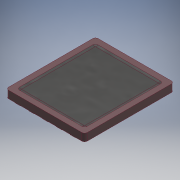
# Autodesk Inventor part: Semiconductor_RadiationDiode
Saved by Autodesk Inventor 2017 (Build 210142000, 142)
## iProperties
Created: 2018-01-16
Part Number: Semiconductor_RadiationDiode
Material: ABS Plastic
Document SubType Name: Modeling
Designer: Bradley
Mass: 0.33228 g
Surface Area: 5.66161 cm^2
Volume: 0.313472 cm^3
Density: 1.06 g/cm^3
Appearance: Smooth - Dark Maroon
Stock Number: X100-7 SMD
Author: Bradley
Autodesk Inventor part; units mm, degrees
ref_plane "YZ Plane" through (0, 0, 0) normal (1, 0, 0) x (0, 1, 0)
ref_plane "XZ Plane" through (0, 0, 0) normal (0, 1, 0) x (-1, 0, 0)
ref_plane "XY Plane" through (0, 0, 0) normal (0, 0, 1) x (1, 0, 0)
sketch "Sketch1" plane through (0, 0, 0) normal (0, 0, 1) x (1, 0, 0)
  line L0 (-7.25, -8.25) -> (7.25, -8.25)
  line L1 (7.25, -8.25) -> (7.25, 8.25)
  line L2 (7.25, 8.25) -> (-7.25, 8.25)
  line L3 (-7.25, 8.25) -> (-7.25, -8.25)
  line L4 (-7.25, -8.25) -> (7.25, 8.25) construction
  line L5 (7.25, -8.25) -> (-7.25, 8.25) construction
  point P0 (0, 0)
  dimension "d0" = 14.5
  dimension "d1" = 16.5
  constraints: 12 end point, 2 midpoint, 2 parallel, 1 horizontal, 1 perpendicular
  measures "d0" distance of L2.end L1.end
  measures "d1" distance of L1.end L0.end
extrude "Extrusion1" add sketch "Sketch1" along normal mid plane 1.38
fillet "Fillet1" radius 0.5 4 edges at (-7.25, 8.25, 0) (7.25, 8.25, 0) (7.25, -8.25, 0) (-7.25, -8.25, 0)
sketch "Sketch2" plane through (0, 0, 0.69) normal (0, 0, 1) x (1, 0, 0)
  arc A0 (-7.25, -7.75) -> (-6.75, -8.25) centre (-6.75, -7.75) ccw projected
  line L0 (-6.75, -8.25) -> (6.75, -8.25) projected
  arc A1 (6.75, -8.25) -> (7.25, -7.75) centre (6.75, -7.75) ccw projected
  line L1 (7.25, -7.75) -> (7.25, 7.75) projected
  arc A2 (7.25, 7.75) -> (6.75, 8.25) centre (6.75, 7.75) ccw projected
  line L2 (6.75, 8.25) -> (-6.75, 8.25) projected
  arc A3 (-6.75, 8.25) -> (-7.25, 7.75) centre (-6.75, 7.75) ccw projected
  line L3 (-7.25, 7.75) -> (-7.25, -7.75) projected
  line L4 (5.75, -7.25) -> (-5.75, -7.25)
  line L5 (-6.25, -6.75) -> (-6.25, 6.75)
  line L6 (-5.75, 7.25) -> (5.75, 7.25)
  line L7 (6.25, 6.75) -> (6.25, -6.75)
  line L8 (6.25, -7.25) -> (-6.25, 7.25) construction
  line L9 (-6.25, -7.25) -> (6.25, 7.25) construction
  arc A4 (-5.75, 7.25) -> (-6.25, 6.75) centre (-5.75, 6.75) ccw
  arc A5 (6.25, 6.75) -> (5.75, 7.25) centre (5.75, 6.75) ccw
  arc A6 (5.75, -7.25) -> (6.25, -6.75) centre (5.75, -6.75) ccw
  arc A7 (-6.25, -6.75) -> (-5.75, -7.25) centre (-5.75, -6.75) ccw
  point P0 (0, 0)
  dimension "d5" = 1
  dimension "d6" = 1
  dimension "d7" = 0.5
  constraints: 12 end point, 8 point on circle, 8 point on line, 8 tangent, 4 centre point, 3 equal radius, 2 midpoint, 2 parallel, 1 horizontal, 1 perpendicular
  measures "d5" distance between parallel lines of L6 L2
  measures "d6" distance between parallel lines of L3 L5
  measures "d7" radius of A4
extrude "Extrusion2" cut sketch "Sketch2" against normal blind 0.1 contours L4 A7 L5 A4 L6 A5 L7 A6
fillet "Fillet2" radius 1 8 edges at (-6.25, 0, 0.59) (-6.1036, 7.1036, 0.59) (0, 7.25, 0.59) (6.1036, 7.1036, 0.59) (6.25, 0, 0.59) (6.1036, -7.1036, 0.59) (0, -7.25, 0.59) (-6.1036, -7.1036, 0.59)
sketch "Sketch3" plane through (0, 0, -0.69) normal (0, 0, -1) x (-1, 0, 0)
  arc A0 (6.75, -8.25) -> (7.25, -7.75) centre (6.75, -7.75) ccw projected
  line L0 (7.25, -7.75) -> (7.25, 7.75) projected
  arc A1 (7.25, 7.75) -> (6.75, 8.25) centre (6.75, 7.75) ccw projected
  line L1 (6.75, 8.25) -> (-6.75, 8.25) projected
  arc A2 (-6.75, 8.25) -> (-7.25, 7.75) centre (-6.75, 7.75) ccw projected
  line L2 (-7.25, 7.75) -> (-7.25, -7.75) projected
  arc A3 (-7.25, -7.75) -> (-6.75, -8.25) centre (-6.75, -7.75) ccw projected
  line L3 (-6.75, -8.25) -> (6.75, -8.25) projected
  line L4 (-5.58, 8.25) -> (-4.58, 8.25)
  line L5 (-4.58, 8.25) -> (-4.58, 6.45)
  line L6 (-4.58, 6.45) -> (-5.58, 6.45)
  line L7 (-5.58, 6.45) -> (-5.58, 8.25)
  line L8 (-3.04, 8.25) -> (-2.04, 8.25)
  line L9 (-2.04, 8.25) -> (-2.04, 6.45)
  line L10 (-2.04, 6.45) -> (-3.04, 6.45)
  line L11 (-3.04, 6.45) -> (-3.04, 8.25)
  line L12 (-0.5, 8.25) -> (0.5, 8.25)
  line L13 (0.5, 8.25) -> (0.5, 6.45)
  line L14 (0.5, 6.45) -> (-0.5, 6.45)
  line L15 (-0.5, 6.45) -> (-0.5, 8.25)
  line L16 (2.04, 8.25) -> (3.04, 8.25)
  line L17 (3.04, 8.25) -> (3.04, 6.45)
  line L18 (3.04, 6.45) -> (2.04, 6.45)
  line L19 (2.04, 6.45) -> (2.04, 8.25)
  line L20 (4.58, 8.25) -> (5.58, 8.25)
  line L21 (5.58, 8.25) -> (5.58, 6.45)
  line L22 (5.58, 6.45) -> (4.58, 6.45)
  line L23 (4.58, 6.45) -> (4.58, 8.25)
  line L24 (-7.25, -7.75) -> (-7.25, 7.75) construction
  line L25 (-7.25, 0) -> (7.25, 0) construction
  line L26 (-5.58, -8.25) -> (-4.58, -8.25)
  line L27 (-4.58, -8.25) -> (-4.58, -6.45)
  line L28 (-4.58, -6.45) -> (-5.58, -6.45)
  line L29 (-5.58, -6.45) -> (-5.58, -8.25)
  line L30 (-3.04, -8.25) -> (-2.04, -8.25)
  line L31 (-2.04, -8.25) -> (-2.04, -6.45)
  line L32 (-2.04, -6.45) -> (-3.04, -6.45)
  line L33 (-3.04, -6.45) -> (-3.04, -8.25)
  line L34 (2.04, -8.25) -> (3.04, -8.25)
  line L35 (3.04, -8.25) -> (3.04, -6.45)
  line L36 (3.04, -6.45) -> (2.04, -6.45)
  line L37 (2.04, -6.45) -> (2.04, -8.25)
  line L38 (4.58, -8.25) -> (5.58, -8.25)
  line L39 (5.58, -8.25) -> (5.58, -6.45)
  line L40 (5.58, -6.45) -> (4.58, -6.45)
  line L41 (4.58, -6.45) -> (4.58, -8.25)
  line L42 (6.75, -8.25) -> (-6.75, -8.25) projected
  line L43 (-0.5, -8.25) -> (0.5, -8.25)
  line L44 (0.5, -8.25) -> (0.5, -5.25)
  line L45 (0.5, -5.25) -> (-0.5, -5.25)
  line L46 (-0.5, -5.25) -> (-0.5, -8.25)
  point P0 (0, 0)
  point P1 (0, 6.45)
  point P2 (0, 0)
  point P3 (0, -5.25)
  dimension "d11" = 1
  dimension "d12" = 1.8
  dimension "d15" = 2.54
  dimension "d20" = 3
  constraints: 82 end point, 16 symmetric about line, 5 midpoint, 4 parallel, 3 horizontal, 2 perpendicular, 2 point on line, 2 vertical alignment, 1 collinear, 32 other
  measures "d11" distance of L5.end L6.end
  measures "d12" distance of L6.end L4.start
  measures "d15" distance of L4.start L8.start
  measures "d20" distance of L43.end L44.end
extrude "Extrusion3" add sketch "Sketch3" along normal blind 0.05 contours L3 L41 L40 L39 | L3 L37 L36 L35 | L21 L22 L23 L1 | L3 L46 L45 L44 | L17 L18 L19 L1 | L3 L33 L32 L31 | L13 L14 L15 L1 | L3 L29 L28 L27 | L9 L10 L11 L1 | L5 L6 L7 L1
equation "\"d6\" = d5"
body "Solid1"
